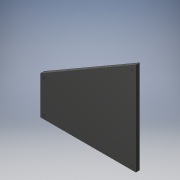
# Autodesk Inventor part: BA10
Saved by Autodesk Inventor 2017 (Build 210142000, 142)
## iProperties
Created: 2018-10-18
Part Number: BA10
Material: ABS Plastic
Document SubType Name: Modeling
Designer: Dell
Density: 1.06 g/cm^3
Appearance: Smooth - Black
Author: Dell
Autodesk Inventor part; units mm, degrees
ref_plane "YZ Plane" through (0, 0, 0) normal (1, 0, 0) x (0, 1, 0)
ref_plane "XZ Plane" through (0, 0, 0) normal (0, 1, 0) x (-1, 0, 0)
ref_plane "XY Plane" through (0, 0, 0) normal (0, 0, 1) x (1, 0, 0)
sketch "Sketch1" plane through (0, 0, 0) normal (0, 0, 1) x (1, 0, 0)
  line L0 (0, 0) -> (505.9426, 0)
  line L1 (505.9426, 0) -> (505.9426, 98.87)
  line L2 (505.9426, 98.87) -> (0, 98.87)
  line L3 (0, 98.87) -> (0, 0)
  line L4 (0, 98.87) -> (252.9713, 244.923)
  line L5 (252.9713, 244.923) -> (505.9426, 98.87)
  point P0 (252.9713, 98.87)
  dimension "d0" = 505.9426
  dimension "d1" = 98.87
  dimension "d2" = 30
  constraints: 12 end point, 2 parallel, 1 horizontal, 1 midpoint, 1 perpendicular, 1 vertical alignment
  measures "d0" distance of L1.end L2.end
  measures "d1" distance of L0.end L1.end
  measures "d2" angle of L2 L5
extrude "Extrusion1" add sketch "Sketch1" along normal blind 10
sketch "Sketch2" plane through (0, 0, 10) normal (0, 0, 1) x (1, 0, 0)
  line L0 (0, 98.87) -> (0, 0) projected
  line L1 (252.9713, 244.923) -> (0, 98.87) projected
  line L2 (505.9426, 98.87) -> (252.9713, 244.923) projected
  line L3 (505.9426, 0) -> (505.9426, 98.87) projected
  line L4 (-10, 0) -> (-10, 104.6435)
  line L5 (-10, 104.6435) -> (252.9713, 256.4701)
  line L6 (252.9713, 256.4701) -> (515.9426, 104.6435)
  line L7 (515.9426, 104.6435) -> (515.9426, 0)
  line L8 (-10, 0) -> (0, 0)
  line L9 (0, 0) -> (505.9426, 0) projected
  line L10 (505.9426, 0) -> (515.9426, 0)
  dimension "d5" = 10
  constraints: 12 end point, 1 collinear, 1 horizontal, 3 other
  measures "d5" distance between parallel lines of L0 L4
extrude "Extrusion2" add sketch "Sketch2" against normal blind 10 contours L0 L8 L4 L5 L6 L7 L10 L3 L2 L1
sketch "Sketch3" plane through (0, 0, 10) normal (0, 0, 1) x (1, 0, 0)
  line L0 (252.9713, 256.4701) -> (515.9426, 104.6435) projected
  line L1 (515.9426, 104.6435) -> (515.9426, 0) projected
  line L2 (252.9713, 256.4701) -> (515.9426, 256.4701)
  line L3 (515.9426, 256.4701) -> (515.9426, 0)
  line L4 (515.9426, 0) -> (252.9713, 0)
  line L5 (252.9713, 0) -> (252.9713, 256.4701)
  point P0 (0, 0)
  constraints: 8 end point, 2 parallel, 1 horizontal, 1 perpendicular
extrude "Extrusion3" cut sketch "Sketch3" against normal through all
sketch "Sketch4" plane through (0, 0, 10) normal (0, 0, 1) x (1, 0, 0)
  line L0 (252.9713, 0) -> (252.9713, 256.4701) construction
  line L1 (252.9713, 256.4701) -> (-10, 104.6435) construction
  line L2 (-10, 104.6435) -> (-10, 0) construction
  line L3 (-10, 0) -> (252.9713, 0) construction
  line L4 (0, 98.87) -> (242.9713, 239.1495) construction
  line L5 (242.9713, 239.1495) -> (242.9713, 10) construction
  line L6 (242.9713, 10) -> (0, 10) construction
  line L7 (0, 10) -> (0, 98.87) construction
  circle A0 centre (0, 10) radius 2.5
  circle A1 centre (0, 98.87) radius 2.5
  circle A2 centre (242.9713, 239.1495) radius 2.5
  circle A3 centre (242.9713, 10) radius 2.5
  point P0 (0, 0)
  dimension "d10" = 10
  dimension "d11" = 5
  dimension "d12" = 5
  dimension "d13" = 5
  dimension "d14" = 5
  constraints: 8 end point, 4 centre point, 4 coincident, 3 other
  measures "d10" distance between parallel lines of L1 L4
  measures "d11" diameter of A0
  measures "d12" diameter of A1
  measures "d13" diameter of A2
  measures "d14" diameter of A3
extrude "Extrusion4" cut sketch "Sketch4" against normal through all
body "Solid1"
